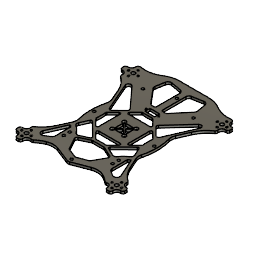
mira_main_body (Autodesk Fusion 360 design; units mm, degrees)
part number: 2026-05-12-18-13-33-373
Autodesk Fusion 360 part; units mm, degrees
(part 1 of 4)
sketch "Esboço1" plane through (0, 0, 0) normal (0, 0, 1) x (1, 0, 0)
  circle A0 centre (75, 87.5) radius 15
  arc A1 (50.5773, 27.2494) -> (51.0282, -29.3922) centre (114.8154, -0.5617) ccw
  line L0 (51.0282, -29.3922) -> (70.7852, -73.1043)
  line L1 (70.4711, 73.2) -> (50.5773, 27.2494)
  circle A2 centre (75, -87.5) radius 15
  circle A3 centre (-75, -87.5) radius 15
  line L2 (-70.4711, 73.2) -> (-50.5773, 27.2494)
  arc A4 (-51.0282, -29.3922) -> (-50.5773, 27.2494) centre (-114.8154, -0.5617) ccw
  line L3 (-51.0282, -29.3922) -> (-70.7852, -73.1043)
  circle A5 centre (-75, 87.5) radius 15
  arc A6 (46.7294, 108.889) -> (73.7447, 102.4474) centre (70.0264, 146.7235) ccw
  arc A7 (-72.6915, 102.3213) -> (-44.7852, 108.3244) centre (-66.5604, 141.6847) ccw
  line L4 (0, 0) -> (0, 132.4678) construction
  arc A8 (-23.7067, 29.0729) -> (-23.5953, 33.2362) centre (-25.8097, 31.2123) ccw
  line L5 (-23.7067, 29.0729) -> (-36.9334, 16.0716)
  arc A9 (-41.7895, 17.0192) -> (-36.9334, 16.0716) centre (-39.0364, 18.2111) ccw
  line L6 (-61.9965, 63.6935) -> (-41.7895, 17.0192)
  line L7 (-55.3948, 68.0303) -> (-23.5953, 33.2362)
  circle A10 centre (-58.3475, 65.3318) radius 4
  arc A11 (9.266, 38.142) -> (7.6383, 38.7303) centre (7.8393, 36.7404) ccw
  line L8 (9.266, 38.142) -> (19.2664, 27.9622)
  arc A12 (17.8415, 24.5606) -> (19.2664, 27.9622) centre (17.8397, 26.5606) ccw
  line L9 (17.8415, 24.5606) -> (-17.871, 24.5283)
  arc A13 (-19.3052, 27.9241) -> (-17.871, 24.5283) centre (-17.8728, 26.5283) ccw
  line L10 (-9.3455, 38.1438) -> (-19.3052, 27.9241)
  arc A14 (-7.7103, 38.7376) -> (-9.3455, 38.1438) centre (-7.9132, 36.7479) ccw
  arc A15 (-7.7103, 38.7376) -> (7.6383, 38.7303) centre (0, 114.3455) ccw
  arc A16 (23.5625, 33.2372) -> (23.6374, 29.1331) centre (25.7596, 31.2246) ccw
  line L11 (23.6374, 29.1331) -> (36.246, 16.5772)
  arc A17 (36.246, 16.5772) -> (41.8922, 17.2564) centre (38.8636, 18.6251) ccw
  line L12 (61.9967, 63.6938) -> (41.8922, 17.2564)
  line L13 (55.4143, 68.0759) -> (23.5625, 33.2372)
  circle A18 centre (58.3695, 65.3802) radius 4
  line L14 (38.1438, -9.3455) -> (27.9241, -19.3052)
  arc A19 (38.1438, -9.3455) -> (38.7376, -7.7103) centre (36.7479, -7.9132) ccw
  arc A20 (38.7303, 7.6383) -> (38.7376, -7.7103) centre (114.3455, 0) ccw
  arc A21 (38.7303, 7.6383) -> (38.142, 9.266) centre (36.7404, 7.8393) ccw
  line L15 (38.142, 9.266) -> (27.9622, 19.2664)
  arc A22 (27.9622, 19.2664) -> (24.5607, 17.8415) centre (26.5606, 17.8397) ccw
  arc A23 (24.5283, -17.871) -> (27.9241, -19.3052) centre (26.5283, -17.8728) ccw
  line L16 (24.5606, 17.8415) -> (24.5283, -17.871)
  arc A24 (19.3052, -27.9241) -> (17.871, -24.5283) centre (17.8728, -26.5283) ccw
  line L17 (9.3455, -38.1438) -> (19.3052, -27.9241)
  arc A25 (7.7103, -38.7376) -> (9.3455, -38.1438) centre (7.9132, -36.7479) ccw
  arc A26 (7.7103, -38.7376) -> (-7.6383, -38.7303) centre (0, -114.3455) ccw
  arc A27 (-9.266, -38.142) -> (-7.6383, -38.7303) centre (-7.8393, -36.7404) ccw
  line L18 (-9.266, -38.142) -> (-19.2664, -27.9622)
  arc A28 (-17.8415, -24.5606) -> (-19.2664, -27.9622) centre (-17.8397, -26.5606) ccw
  line L19 (-17.8415, -24.5606) -> (17.871, -24.5283)
  arc A29 (-27.9955, -19.2498) -> (-24.5916, -17.8264) centre (-26.5916, -17.8253) ccw
  line L20 (-38.1463, -9.2454) -> (-27.9955, -19.2498)
  arc A30 (-38.7321, -7.6192) -> (-38.1463, -9.2454) centre (-36.7424, -7.821) ccw
  arc A31 (-38.7321, -7.6192) -> (-38.7256, 7.6527) centre (-114.3432, 0.0492) ccw
  arc A32 (-38.1376, 9.2791) -> (-38.7256, 7.6527) centre (-36.7356, 7.8528) ccw
  line L21 (-38.1376, 9.2791) -> (-27.9736, 19.2699)
  arc A33 (-24.5716, 17.8424) -> (-27.9736, 19.2699) centre (-26.5716, 17.8436) ccw
  line L22 (-24.5716, 17.8424) -> (-24.5916, -17.8264)
  arc A34 (-34.7856, -45.3775) -> (-28.3187, -47.4234) centre (-30.444, -42.8975) ccw
  arc A35 (-34.7856, -45.3775) -> (-44.4886, -35.8486) centre (-56.4937, -57.7776) ccw
  arc A36 (-46.6438, -29.4035) -> (-44.4886, -35.8486) centre (-42.0875, -31.4628) ccw
  line L23 (-40.6601, -16.1647) -> (-46.6438, -29.4035)
  arc A37 (-37.4337, -15.5639) -> (-40.6601, -16.1647) centre (-38.8376, -16.9884) ccw
  line L24 (-37.4337, -15.5639) -> (-14.6425, -38.0264)
  arc A38 (-15.1963, -41.2612) -> (-14.6425, -38.0264) centre (-16.0464, -39.4508) ccw
  line L25 (-15.1963, -41.2612) -> (-28.3187, -47.4234)
  arc A39 (44.339, -36.0244) -> (34.6129, -45.4956) centre (56.2565, -57.9923) ccw
  arc A40 (44.339, -36.0244) -> (46.7322, -29.5993) centre (42.0339, -31.5075) ccw
  line L26 (40.9054, -16.7074) -> (46.7322, -29.5993)
  arc A41 (40.9054, -16.7074) -> (37.3489, -15.6517) centre (38.8619, -17.0732) ccw
  line L27 (37.3489, -15.6517) -> (14.46, -38.0146)
  arc A42 (14.46, -38.0146) -> (14.9942, -41.2515) centre (15.8549, -39.4469) ccw
  arc A43 (28.1234, -47.5076) -> (34.6129, -45.4956) centre (30.28, -42.9921) ccw
  line L28 (14.9942, -41.2515) -> (28.1234, -47.5076)
  line L29 (-9.1318, 102.3881) -> (-26.9725, 105.5339)
  arc A44 (-26.9725, 105.5339) -> (-32.7648, 101.4781) centre (-27.8408, 100.6098) ccw
  line L30 (-32.7648, 101.4781) -> (-35.4243, 86.3954)
  arc A45 (-35.4243, 86.3954) -> (-34.3305, 82.3132) centre (-30.5003, 85.5271) ccw
  line L31 (-34.3305, 82.3132) -> (-14.3032, 58.4456)
  arc A46 (-14.3032, 58.4456) -> (-10.473, 56.6595) centre (-10.473, 61.6595) ccw
  line L32 (-10.473, 56.6595) -> (-7, 56.6595)
  arc A47 (-7, 56.6595) -> (-5, 58.6595) centre (-7, 58.6595) ccw
  arc A48 (-5, 97.464) -> (-9.1318, 102.3881) centre (-10, 97.464) ccw
  line L33 (-5, 58.6595) -> (-5, 97.464)
  arc A49 (9.1318, 102.3881) -> (5, 97.464) centre (10, 97.464) ccw
  line L34 (9.1318, 102.3881) -> (26.9725, 105.5339)
  arc A50 (32.7648, 101.4781) -> (26.9725, 105.5339) centre (27.8408, 100.6098) ccw
  line L35 (32.7648, 101.4781) -> (35.4243, 86.3954)
  arc A51 (34.3305, 82.3132) -> (35.4243, 86.3954) centre (30.5003, 85.5271) ccw
  line L36 (34.3305, 82.3132) -> (14.3032, 58.4456)
  arc A52 (10.473, 56.6595) -> (14.3032, 58.4456) centre (10.473, 61.6595) ccw
  line L37 (10.473, 56.6595) -> (7, 56.6595)
  arc A53 (5, 58.6595) -> (7, 56.6595) centre (7, 58.6595) ccw
  line L38 (5, 58.6595) -> (5, 97.464)
  line L39 (0, 0) -> (0, 114.3455) construction
  line L40 (2.1213, -0.7071) -> (8.1464, -6.7322)
  line L41 (0, 0) -> (20, 0) construction
  circle A54 centre (10, 10) radius 1.5
  line L42 (-10, -10) -> (10, 10) construction
  line L43 (-2.1213, 0.7071) -> (-8.1464, 6.7322)
  arc A55 (-6.7322, -8.1464) -> (-6.3787, -9) centre (-6.3787, -8.5) ccw
  arc A56 (-6.3787, 9) -> (-6.7322, 8.1464) centre (-6.3787, 8.5) ccw
  arc A57 (-0.7071, 2.1213) -> (0.7071, 2.1213) centre (0, 2.8284) ccw
  line L44 (8.1464, 6.7322) -> (2.1213, 0.7071)
  line L45 (6.7322, -8.1464) -> (0.7071, -2.1213)
  arc A58 (6.3787, -9) -> (6.7322, -8.1464) centre (6.3787, -8.5) ccw
  line L46 (-8.1464, -6.7322) -> (-2.1213, -0.7071)
  line L47 (-10, 10) -> (10, 10)
  line L48 (-0.7071, -2.1213) -> (-6.7322, -8.1464)
  line L49 (-9, 6.3787) -> (-9, -6.3787)
  line L50 (10, -10) -> (-10, -10)
  circle A59 centre (-10, 10) radius 1.5
  line L51 (10, 10) -> (10, -10)
  arc A60 (6.7322, 8.1464) -> (6.3787, 9) centre (6.3787, 8.5) ccw
  arc A61 (9, 6.3787) -> (8.1464, 6.7322) centre (8.5, 6.3787) ccw
  arc A62 (0.7071, -2.1213) -> (-0.7071, -2.1213) centre (0, -2.8284) ccw
  arc A63 (2.1213, 0.7071) -> (2.1213, -0.7071) centre (2.8284, 0) ccw
  arc A64 (-2.1213, -0.7071) -> (-2.1213, 0.7071) centre (-2.8284, 0) ccw
  arc A65 (8.1464, -6.7322) -> (9, -6.3787) centre (8.5, -6.3787) ccw
  circle A66 centre (10, -10) radius 1.5
  arc A67 (-9, -6.3787) -> (-8.1464, -6.7322) centre (-8.5, -6.3787) ccw
  line L52 (-10, -10) -> (-10, 10)
  line L53 (-6.3787, -9) -> (6.3787, -9)
  line L54 (10, -10) -> (-10, 10) construction
  line L55 (-6.7322, 8.1464) -> (-0.7071, 2.1213)
  line L56 (0.7071, 2.1213) -> (6.7322, 8.1464)
  line L57 (9, -6.3787) -> (9, 6.3787)
  circle A68 centre (-10, -10) radius 1.5
  line L58 (6.3787, 9) -> (-6.3787, 9)
  arc A69 (-8.1464, 6.7322) -> (-9, 6.3787) centre (-8.5, 6.3787) ccw
  circle A70 centre (0, -87.5) radius 6
  line L59 (0, -87.5) -> (0, -54) construction
  line L60 (0, -81.5) -> (-15.6612, -75.3836)
  line L61 (0, -81.5) -> (16.4256, -75.2214)
  line L62 (2.1423, -93.1045) -> (36.9275, -79.8081)
  line L63 (-2.1827, -93.0889) -> (-35.9657, -79.8952)
  arc A71 (-35.9657, -79.8952) -> (-60.1979, -89.9288) centre (0.31, -201.7835) ccw
  arc A72 (60.2098, -89.9999) -> (36.9275, -79.8081) centre (-2.2046, -200.8918) ccw
  circle A73 centre (0, -87.5) radius 2.15
  line L64 (-26.2105, -50.915) -> (-10.6059, -43.5872)
  line L65 (-9.3307, -43.3027) -> (9.3218, -43.3027)
  line L66 (10.6123, -43.5944) -> (26.8632, -51.3381)
  line L67 (28.1945, -55.5044) -> (17.9762, -73.8773)
  line L68 (-17.2021, -74.0283) -> (-27.5676, -55.0697)
  arc A74 (-26.2105, -50.915) -> (-27.5676, -55.0697) centre (-24.9353, -53.6305) ccw
  arc A75 (-9.3307, -43.3027) -> (-10.6059, -43.5872) centre (-9.3307, -46.3027) ccw
  arc A76 (10.6123, -43.5944) -> (9.3218, -43.3027) centre (9.3218, -46.3027) ccw
  arc A77 (28.1945, -55.5044) -> (26.8632, -51.3381) centre (25.5727, -54.0463) ccw
  arc A78 (16.4256, -75.2214) -> (17.9762, -73.8773) centre (15.3544, -72.4192) ccw
  arc A79 (-17.2021, -74.0283) -> (-15.6612, -75.3836) centre (-14.5698, -72.5892) ccw
  line L69 (25.7561, 114.8285) -> (-22.9214, 114.8285)
  arc A80 (46.7294, 108.889) -> (25.7561, 114.8285) centre (25.7561, 74.8285) ccw
  arc A81 (-22.9214, 114.8285) -> (-44.7852, 108.3244) centre (-22.9214, 74.8285) ccw
  point P0 (9, 7.5858)
  point P1 (9, -7.5858)
  point P2 (-10, -43.3027)
  point P3 (10, -43.3027)
  dimension "d1" = 30
  dimension "d2" = 30
  dimension "d3" = 30
  dimension "d4" = 30
  dimension "d5" = 127.25
  dimension "d6" = 70
  dimension "d9" = 150
  dimension "d10" = 150
  dimension "d11" = 8
  dimension "d12" = 3
  dimension "d13" = 4
  dimension "d14" = 2
  dimension "d15" = 4
  dimension "d16" = 2
  dimension "d17" = 69.738
  dimension "d18" = 69.738
  dimension "d19" = 32
  dimension "d20" = 25
  dimension "d21" = 5
  dimension "d22" = 4
  dimension "d23" = 4
  dimension "d24" = 4
  dimension "d25" = 4
  dimension "d26" = 130
  dimension "d27" = 100
  dimension "d28" = 5
  dimension "d29" = 2
  dimension "d30" = 38.8045
  dimension "d31" = 31.1569
  dimension "d32" = 15.0827
  dimension "d33" = 17.8408
  dimension "d34" = 5
  dimension "d35" = 100
  dimension "d36" = 2
  dimension "d37" = 5
  dimension "d38" = 3.473
  dimension "d39" = 31.1569
  dimension "d40" = 38.8045
  dimension "d41" = 17.8408
  dimension "d42" = 5
  dimension "d43" = 15.0827
  dimension "d44" = 5
  dimension "d45" = 5
  dimension "d62" = 360
  dimension "d63" = 3
  dimension "d64" = 3
  dimension "d65" = 3
  dimension "d66" = 3
  dimension "d67" = 1
  dimension "d68" = 1
  dimension "d69" = 1
  dimension "d70" = 0.5
  dimension "d71" = 20
  dimension "d72" = 20
  dimension "d73" = 1
  dimension "d149" = 12
  dimension "d150" = 87.5
  dimension "d153" = 4.3
  dimension "d166" = 140
  dimension "d167" = 140
  dimension "d168" = 20
  dimension "d169" = 4
  dimension "d170" = 3
  dimension "d171" = 40
  dimension "d173" = 87.5
  dimension "d186" = 87.5
  dimension "d187" = 87.5
  dimension "d188" = 87.5
  dimension "d189" = 75
  dimension "d190" = 75
  constraint coincident L2.start A5
  constraint coincident L3.end A3
  constraint coincident A72.start A2
  constraint coincident A71.end A3
  constraint tangent L2 A4
  constraint tangent A4 L3
  constraint tangent A1 L1
  constraint tangent A1 L0
  constraint equal A1 A4
  constraint coincident L1.start A0
  constraint equal L1 L2
  constraint equal L0 L3
  constraint coincident A7.start A5
  constraint coincident A6.end A0
  constraint tangent A5 A7
  constraint tangent A0 A6
  constraint coincident L4.start L39.start
  constraint symmetric A0 A5 L4
  constraint symmetric A2 A3 L4
  constraint symmetric A1 A4 L4
  constraint coincident L6.start A10
  constraint coincident L7.start A10
  constraint tangent A9 L6
  constraint tangent L5 A9
  constraint tangent A8 L7
  constraint tangent A8 L5
  constraint equal A8 A9
  constraint tangent L7 A10
  constraint parallel L5 L21
  constraint tangent L21 A33
  constraint tangent A33 L22
  constraint tangent A29 L20
  constraint tangent A29 L22
  constraint equal A29 A33
  constraint tangent L20 A30
  constraint tangent A30 A31
  constraint equal A30 A33
  constraint tangent A32 L21
  constraint tangent A31 A32
  constraint equal A32 A33
  constraint equal L20 L21
  constraint parallel L20 L24
  constraint tangent A37 L24
  constraint tangent L23 A37
  constraint tangent L24 A38
  constraint tangent A38 L25
  constraint equal A37 A38
  constraint tangent A34 L25
  constraint tangent A34 A35
  constraint tangent A36 L23
  constraint tangent A35 A36
  constraint equal A34 A36
  constraint perpendicular L32 L33
  constraint perpendicular L29 L30
  constraint tangent A44 L30
  constraint tangent L29 A44
  constraint tangent A48 L33
  constraint tangent L29 A48
  constraint equal A44 A48
  constraint tangent L30 A45
  constraint tangent A45 L31
  constraint equal A44 A45
  constraint tangent L31 A46
  constraint tangent A46 L32
  constraint equal A44 A46
  constraint tangent L32 A47
  constraint tangent A47 L33
  constraint coincident A15.centre L39.end
  constraint coincident L0.end A2
  constraint coincident L13.start A18
  constraint coincident L12.start A18
  constraint horizontal L50
  constraint perpendicular L50 L52
  constraint parallel L47 L50
  constraint parallel L51 L52
  constraint coincident L4.start L54
  constraint coincident L4.start L42
  constraint coincident L50.start L51.end
  constraint coincident L42.start L50.end
  constraint coincident A54.centre L42.end
  constraint coincident L47.start A59.centre
  constraint parallel L51 L57
  constraint parallel L40 L54
  constraint parallel L42 L44
  constraint perpendicular L41 L57
  constraint coincident P1 L57
  constraint coincident P1 L40
  constraint tangent A65 L57
  constraint tangent L40 A65
  constraint coincident P0 L57
  constraint coincident P0 L44
  constraint tangent A61 L57
  constraint tangent L44 A61
  constraint equal A61 A65
  constraint tangent L44 A63
  constraint tangent L40 A63
  constraint coincident A70.centre L59.start
  constraint vertical L59
  constraint coincident A70 L60.start
  constraint coincident L59 L60.start
  constraint coincident A70 L62.start
  constraint coincident A70 L63.start
  constraint tangent A70 L63
  constraint tangent A70 L62
  constraint parallel L60 L63
  constraint parallel L61 L62
  constraint concentric A70 A73
  constraint horizontal L65
  constraint parallel L25 L64
  constraint parallel L28 L66
  constraint symmetric L59 P2 P3
  constraint tangent L64 A74
  constraint tangent L68 A74
  constraint coincident P2 L64
  constraint tangent L64 A75
  constraint tangent L65 A75
  constraint equal A74 A75
  constraint coincident P3 L65
  constraint coincident P3 L66
  constraint tangent L65 A76
  constraint tangent L66 A76
  constraint equal A74 A76
  constraint tangent L66 A77
  constraint tangent L67 A77
  constraint equal A74 A77
  constraint tangent L61 A78
  constraint tangent L67 A78
  constraint equal A74 A78
  constraint tangent L60 A79
  constraint tangent L68 A79
  constraint equal A74 A79
  constraint perpendicular L4 L69
  constraint tangent L69 A80
  constraint tangent A6 A80
  constraint tangent L69 A81
  constraint tangent A7 A81
  constraint equal A80 A81
  measures "d1" diameter of A5
  measures "d2" diameter of A0
  measures "d3" diameter of A3
  measures "d4" diameter of A2
  measures "d5" radius of A72
  measures "d6" radius of A4
  measures "d9" distance of A3.centre A2.centre
  measures "d10" distance of A5.centre A0.centre
  measures "d11" diameter of A10
  measures "d12" radius of A9
  measures "d13" distance of L5 L21
  measures "d14" radius of A33
  measures "d15" distance of L20 L24
  measures "d16" radius of A37
  measures "d17" angle of L23 L24
  measures "d18" angle of L24 L25
  measures "d19" distance of L24.end A37.start
  measures "d20" radius of A35
  measures "d21" radius of A34
  measures "d22" distance of L2 L6
  measures "d23" distance of L1 L12
  measures "d24" distance of L0 L26
  measures "d25" distance of L3 L23
  measures "d26" angle of L31 L32
  measures "d27" angle of L29 L33
  measures "d28" radius of A44
  measures "d29" radius of A47
  measures "d30" distance of A48.start A47.end
  measures "d31" distance of L31.end A45.end
  measures "d32" vertical distance of A44.end L30.end
  measures "d33" horizontal distance of L29.start L29.end
  measures "d34" distance of L33 L39
  measures "d35" angle of L34 L38
  measures "d36" radius of A53
  measures "d37" radius of A52
  measures "d38" distance of A52.start L37.end
  measures "d39" distance of A51.start L36.end
  measures "d40" distance of A49.end A53.start
  measures "d41" horizontal distance of A49.start L34.end
  measures "d42" radius of A50
  measures "d43" vertical distance of L35.end A50.start
  measures "d44" radius of A51
  measures "d45" distance of L38 L39
  measures "d63" diameter of A66
  measures "d64" diameter of A68
  measures "d65" diameter of A54
  measures "d66" diameter of A59
  measures "d67" distance of L51 L57
  measures "d68" distance of L42 L44
  measures "d69" distance of L40 L54
  measures "d70" radius of A65
  measures "d71" distance of L50.start A54.centre
  measures "d72" distance of L42.start L50.start
  measures "d73" radius of A63
  measures "d149" diameter of A70
  measures "d150" distance of L4.start A70.centre
  measures "d153" diameter of A73
  measures "d166" angle of L61 L67
  measures "d167" angle of L60 L68
  measures "d168" distance of P2 P3
  measures "d169" distance of L28 L66
  measures "d170" radius of A74
  measures "d171" radius of A80
  measures "d173" vertical distance of A2.centre L4.start
  measures "d186" vertical distance of A0.centre L4.start
  measures "d187" vertical distance of A5.centre L4.start
  measures "d188" vertical distance of A3.centre L4.start
  measures "d189" horizontal distance of L4.start A3.centre
  measures "d190" horizontal distance of A0.centre L4.start
extrude "Extrusão1" add sketch "Esboço1" along normal mid plane 4 contours A0 | A0 A1 L0 L1 A2 A3 L2 A4 L3 A5 A6 A7 A70 L62 L63 A71 A72 L69 A80 A81 | A2 | A5 | A70 | A3 | A54 L47 L51 | A54 L47 L51 | A54 L47 L50 A59 L51 A66 L52 A68 | L47 A59 L52 | L47 A59 L52 | L50 L51 A66 | L50 L51 A66 | L50 L52 A68 | L50 L52 A68
sketch "Esboço2" plane through (0, 0, 2) normal (0, 0, 1) x (-1, 0, 0)
  line L0 (14.9943, 41.2512) -> (28.1237, 47.5069)
  line L1 (49.5538, 39.7214) -> (47.4521, 41.7697)
  arc A0 (47.15, 42.4858) -> (47.4521, 41.7697) centre (48.15, 42.4858) ccw
  arc A1 (49.5538, 39.7214) -> (51.1653, 40.0309) centre (50.2517, 40.4376) ccw
  line L2 (47.15, 42.4858) -> (47.15, 67.561)
  arc A2 (49.4611, 71.7764) -> (47.15, 67.561) centre (52.15, 67.561) ccw
  arc A3 (-14.4588, 38.0133) -> (-14.9943, 41.2512) centre (-15.8546, 39.4456) ccw
  arc A4 (-47.15, 67.561) -> (-49.4611, 71.7764) centre (-52.15, 67.561) ccw
  circle A5 centre (-40.65, 60) radius 2.15
  arc A6 (-24.5283, 17.871) -> (-27.9241, 19.3052) centre (-26.5283, 17.8728) ccw
  arc A7 (-47.4521, 41.7697) -> (-47.15, 42.4858) centre (-48.15, 42.4858) ccw
  line L3 (-47.15, 42.4858) -> (-47.15, 67.561)
  line L4 (-28.1237, 47.5069) -> (-14.9943, 41.2512)
  line L5 (-32.8675, 14.4875) -> (-27.9241, 19.3052)
  line L6 (-49.4611, 71.7764) -> (-57.5607, 76.943)
  arc A8 (14.9943, 41.2512) -> (14.4588, 38.0133) centre (15.8546, 39.4456) ccw
  arc A9 (34.6056, 45.4913) -> (44.3323, 36.0121) centre (56.2613, 57.9825) ccw
  line L7 (-49.5538, 39.7214) -> (-47.4521, 41.7697)
  arc A10 (-40.5988, 16.2982) -> (-37.3758, 15.6793) centre (-38.7717, 17.1116) ccw
  arc A11 (-57.5607, 76.943) -> (-64.8173, 70.6939) centre (-60.2496, 72.7276) ccw
  arc A12 (-28.1237, 47.5069) -> (-34.6056, 45.4913) centre (-30.2744, 42.9931) ccw
  line L8 (-14.4588, 38.0133) -> (-15.8157, 36.6909)
  line L9 (17.8415, 24.5606) -> (-17.871, 24.5283)
  circle A13 centre (-40.65, 50) radius 2.15
  line L10 (-19.3052, 27.9241) -> (-9.3455, 38.1438)
  arc A14 (-7.7103, 38.7376) -> (-9.3455, 38.1438) centre (-7.9132, 36.7479) ccw
  arc A15 (-7.7103, 38.7376) -> (7.6383, 38.7303) centre (0, 114.3455) ccw
  arc A16 (-19.3052, 27.9241) -> (-17.871, 24.5283) centre (-17.8728, 26.5283) ccw
  arc A17 (-51.1653, 40.0309) -> (-49.5538, 39.7214) centre (-50.2517, 40.4376) ccw
  circle A18 centre (40.65, 50) radius 2.15
  circle A19 centre (40.65, 60) radius 2.15
  line L11 (49.4611, 71.7764) -> (57.5607, 76.943)
  arc A20 (34.6056, 45.4913) -> (28.1237, 47.5069) centre (30.2744, 42.9931) ccw
  arc A21 (9.266, 38.142) -> (7.6383, 38.7303) centre (7.8393, 36.7404) ccw
  arc A22 (-38.1438, 9.3455) -> (-38.7376, 7.7103) centre (-36.7479, 7.9132) ccw
  arc A23 (64.8173, 70.6939) -> (57.5607, 76.943) centre (60.2496, 72.7276) ccw
  line L12 (51.1653, 40.0309) -> (64.8173, 70.6939)
  arc A24 (-38.7376, -7.7103) -> (-38.7303, -7.6383) centre (-114.3455, 0) ccw
  arc A25 (46.5142, 29.5844) -> (44.3323, 36.0121) centre (41.9465, 31.618) ccw
  line L13 (-51.1653, 40.0309) -> (-64.8173, 70.6939)
  line L14 (0, 38.3455) -> (0, 95) construction
  line L15 (19.3052, -27.9241) -> (9.3455, -38.1438)
  arc A26 (7.7103, -38.7376) -> (9.3455, -38.1438) centre (7.9132, -36.7479) ccw
  arc A27 (7.7103, -38.7376) -> (-7.6383, -38.7303) centre (0, -114.3455) ccw
  arc A28 (-9.266, -38.142) -> (-7.6383, -38.7303) centre (-7.8393, -36.7404) ccw
  line L16 (-9.266, -38.142) -> (-19.2664, -27.9622)
  arc A29 (-17.8415, -24.5606) -> (-19.2664, -27.9622) centre (-17.8397, -26.5606) ccw
  line L17 (-17.8415, -24.5606) -> (17.871, -24.5283)
  arc A30 (19.3052, -27.9241) -> (17.871, -24.5283) centre (17.8728, -26.5283) ccw
  line L18 (70.4711, -73.2) -> (50.5773, -27.2494)
  arc A31 (51.0282, 29.3922) -> (50.5773, -27.2494) centre (114.8154, 0.5617) ccw
  line L19 (51.0282, 29.3922) -> (70.7852, 73.1043)
  arc A32 (70.7852, 73.1043) -> (60.1979, 89.9288) centre (75, 87.5) ccw
  arc A33 (35.9657, 79.8952) -> (60.1979, 89.9288) centre (-0.31, 201.7835) ccw
  arc A34 (-60.2098, 89.9999) -> (-70.7852, 73.1043) centre (-75, 87.5) ccw
  line L20 (-70.7852, 73.1043) -> (-51.0282, 29.3922)
  arc A35 (-50.5773, -27.2494) -> (-51.0282, 29.3922) centre (-114.8154, 0.5617) ccw
  line L21 (-50.5773, -27.2494) -> (-70.4711, -73.2)
  arc A36 (-70.4711, -73.2) -> (-73.7447, -102.4474) centre (-75, -87.5) ccw
  arc A37 (-46.7294, -108.889) -> (-73.7447, -102.4474) centre (-70.0264, -146.7235) ccw
  arc A38 (72.6915, -102.3213) -> (44.7852, -108.3244) centre (66.5604, -141.6847) ccw
  arc A39 (72.6915, -102.3213) -> (70.4711, -73.2) centre (75, -87.5) ccw
  arc A40 (38.1376, -9.2791) -> (38.7256, -7.6527) centre (36.7356, -7.8528) ccw
  line L22 (38.1376, -9.2791) -> (27.9736, -19.2699)
  arc A41 (24.5716, -17.8424) -> (27.9736, -19.2699) centre (26.5716, -17.8436) ccw
  line L23 (24.5716, -17.8424) -> (24.5916, 17.8264)
  arc A42 (27.9955, 19.2498) -> (24.5916, 17.8264) centre (26.5916, 17.8253) ccw
  line L24 (27.9955, 19.2498) -> (38.1463, 9.2454)
  arc A43 (38.7321, 7.6192) -> (38.1463, 9.2454) centre (36.7424, 7.821) ccw
  arc A44 (38.7321, 7.6192) -> (38.7256, -7.6527) centre (114.3432, -0.0492) ccw
  arc A45 (-10.473, -56.6595) -> (-14.3032, -58.4456) centre (-10.473, -61.6595) ccw
  line L25 (-10.473, -56.6595) -> (-7, -56.6595)
  arc A46 (-5, -58.6595) -> (-7, -56.6595) centre (-7, -58.6595) ccw
  line L26 (-5, -58.6595) -> (-5, -97.464)
  arc A47 (-9.1318, -102.3881) -> (-5, -97.464) centre (-10, -97.464) ccw
  line L27 (-9.1318, -102.3881) -> (-26.9725, -105.5339)
  arc A48 (-32.7648, -101.4781) -> (-26.9725, -105.5339) centre (-27.8408, -100.6098) ccw
  line L28 (-32.7648, -101.4781) -> (-35.4243, -86.3954)
  arc A49 (-34.3305, -82.3132) -> (-35.4243, -86.3954) centre (-30.5003, -85.5271) ccw
  line L29 (-34.3305, -82.3132) -> (-14.3032, -58.4456)
  line L30 (5, -97.464) -> (5, -58.6595)
  arc A50 (7, -56.6595) -> (5, -58.6595) centre (7, -58.6595) ccw
  line L31 (7, -56.6595) -> (10.473, -56.6595)
  arc A51 (14.3032, -58.4456) -> (10.473, -56.6595) centre (10.473, -61.6595) ccw
  line L32 (14.3032, -58.4456) -> (34.3305, -82.3132)
  arc A52 (35.4243, -86.3954) -> (34.3305, -82.3132) centre (30.5003, -85.5271) ccw
  line L33 (35.4243, -86.3954) -> (32.7648, -101.4781)
  arc A53 (26.9725, -105.5339) -> (32.7648, -101.4781) centre (27.8408, -100.6098) ccw
  line L34 (26.9725, -105.5339) -> (9.1318, -102.3881)
  arc A54 (5, -97.464) -> (9.1318, -102.3881) centre (10, -97.464) ccw
  arc A55 (-38.7303, -7.6383) -> (-38.142, -9.266) centre (-36.7404, -7.8393) ccw
  arc A56 (-38.7303, -7.6383) -> (-38.7376, 7.7103) centre (-114.3455, 0) ccw
  arc A57 (-38.1438, 9.3455) -> (-38.7376, 7.7103) centre (-36.7479, 7.9132) ccw
  line L35 (-38.1438, 9.3455) -> (-27.9241, 19.3052)
  arc A58 (-24.5283, 17.871) -> (-27.9241, 19.3052) centre (-26.5283, 17.8728) ccw
  line L36 (-24.5283, 17.871) -> (-24.5606, -17.8415)
  arc A59 (-27.9622, -19.2664) -> (-24.5607, -17.8415) centre (-26.5606, -17.8397) ccw
  line L37 (-27.9622, -19.2664) -> (-38.142, -9.266)
  arc A60 (37.4337, 15.5639) -> (40.6601, 16.1647) centre (38.8376, 16.9884) ccw
  line L38 (37.4337, 15.5639) -> (14.6425, 38.0264)
  arc A61 (15.1963, 41.2612) -> (14.6425, 38.0264) centre (16.0464, 39.4508) ccw
  line L39 (15.1963, 41.2612) -> (28.3187, 47.4234)
  arc A62 (34.7856, 45.3775) -> (28.3187, 47.4234) centre (30.444, 42.8975) ccw
  arc A63 (34.7856, 45.3775) -> (44.4886, 35.8486) centre (56.4937, 57.7776) ccw
  arc A64 (46.6438, 29.4035) -> (44.4886, 35.8486) centre (42.0875, 31.4628) ccw
  line L40 (46.6438, 29.4035) -> (40.6601, 16.1647)
  line L41 (41.7895, -17.0192) -> (61.9965, -63.6935)
  arc A65 (55.3948, -68.0303) -> (61.9965, -63.6935) centre (58.3475, -65.3318) ccw
  line L42 (55.3948, -68.0303) -> (23.5953, -33.2362)
  arc A66 (23.7067, -29.0729) -> (23.5953, -33.2362) centre (25.8097, -31.2123) ccw
  line L43 (23.7067, -29.0729) -> (36.9334, -16.0716)
  arc A67 (41.7895, -17.0192) -> (36.9334, -16.0716) centre (39.0364, -18.2111) ccw
  arc A68 (9.266, 38.142) -> (7.6383, 38.7303) centre (7.8393, 36.7404) ccw
  line L44 (9.266, 38.142) -> (19.2664, 27.9622)
  arc A69 (17.8415, 24.5606) -> (19.2664, 27.9622) centre (17.8397, 26.5606) ccw
  line L45 (17.8415, 24.5606) -> (-17.871, 24.5283)
  arc A70 (-19.3052, 27.9241) -> (-17.871, 24.5283) centre (-17.8728, 26.5283) ccw
  line L46 (-19.3052, 27.9241) -> (-9.3455, 38.1438)
  arc A71 (-7.7103, 38.7376) -> (-9.3455, 38.1438) centre (-7.9132, 36.7479) ccw
  arc A72 (-7.7103, 38.7376) -> (7.6383, 38.7303) centre (0, 114.3455) ccw
  arc A73 (-40.9054, 16.7074) -> (-37.3489, 15.6517) centre (-38.8619, 17.0732) ccw
  line L47 (-40.9054, 16.7074) -> (-46.7322, 29.5993)
  arc A74 (-44.339, 36.0244) -> (-46.7322, 29.5993) centre (-42.0339, 31.5075) ccw
  arc A75 (-44.339, 36.0244) -> (-34.6129, 45.4956) centre (-56.2565, 57.9923) ccw
  arc A76 (-28.1234, 47.5076) -> (-34.6129, 45.4956) centre (-30.28, 42.9921) ccw
  line L48 (-28.1234, 47.5076) -> (-14.9942, 41.2515)
  arc A77 (-14.46, 38.0146) -> (-14.9942, 41.2515) centre (-15.8549, 39.4469) ccw
  line L49 (-14.46, 38.0146) -> (-37.3489, 15.6517)
  arc A78 (-61.9967, -63.6938) -> (-55.4143, -68.0759) centre (-58.3695, -65.3802) ccw
  line L50 (-61.9967, -63.6938) -> (-41.8922, -17.2564)
  arc A79 (-36.246, -16.5772) -> (-41.8922, -17.2564) centre (-38.8636, -18.6251) ccw
  line L51 (-36.246, -16.5772) -> (-23.6374, -29.1331)
  arc A80 (-23.5625, -33.2372) -> (-23.6374, -29.1331) centre (-25.7596, -31.2246) ccw
  line L52 (-23.5625, -33.2372) -> (-55.4143, -68.0759)
  line L53 (8.1464, -6.7322) -> (2.1213, -0.7071)
  arc A81 (2.1213, 0.7071) -> (2.1213, -0.7071) centre (2.8284, 0) ccw
  line L54 (2.1213, 0.7071) -> (8.1464, 6.7322)
  arc A82 (9, 6.3787) -> (8.1464, 6.7322) centre (8.5, 6.3787) ccw
  line L55 (9, 6.3787) -> (9, -6.3787)
  arc A83 (8.1464, -6.7322) -> (9, -6.3787) centre (8.5, -6.3787) ccw
  arc A84 (-6.7322, -8.1464) -> (-6.3787, -9) centre (-6.3787, -8.5) ccw
  line L56 (-6.7322, -8.1464) -> (-0.7071, -2.1213)
  arc A85 (0.7071, -2.1213) -> (-0.7071, -2.1213) centre (0, -2.8284) ccw
  line L57 (0.7071, -2.1213) -> (6.7322, -8.1464)
  arc A86 (6.3787, -9) -> (6.7322, -8.1464) centre (6.3787, -8.5) ccw
  line L58 (6.3787, -9) -> (-6.3787, -9)
  arc A87 (-8.1464, 6.7322) -> (-9, 6.3787) centre (-8.5, 6.3787) ccw
  line L59 (-8.1464, 6.7322) -> (-2.1213, 0.7071)
  arc A88 (-2.1213, -0.7071) -> (-2.1213, 0.7071) centre (-2.8284, 0) ccw
  line L60 (-2.1213, -0.7071) -> (-8.1464, -6.7322)
  arc A89 (-9, -6.3787) -> (-8.1464, -6.7322) centre (-8.5, -6.3787) ccw
  line L61 (-9, -6.3787) -> (-9, 6.3787)
  arc A90 (6.7322, 8.1464) -> (6.3787, 9) centre (6.3787, 8.5) ccw
  line L62 (6.7322, 8.1464) -> (0.7071, 2.1213)
  arc A91 (-0.7071, 2.1213) -> (0.7071, 2.1213) centre (0, 2.8284) ccw
  line L63 (-0.7071, 2.1213) -> (-6.7322, 8.1464)
  arc A92 (-6.3787, 9) -> (-6.7322, 8.1464) centre (-6.3787, 8.5) ccw
  line L64 (-6.3787, 9) -> (6.3787, 9)
  line L65 (35.9657, 79.8952) -> (2.1827, 93.0889)
  arc A93 (2.1827, 93.0889) -> (-2.1423, 93.1045) centre (0, 87.5) ccw
  line L66 (0, 81.5) -> (15.6612, 75.3836)
  line L67 (-16.4256, 75.2214) -> (0, 81.5)
  line L68 (-2.1423, 93.1045) -> (-36.9275, 79.8081)
  arc A94 (-60.2098, 89.9999) -> (-36.7745, 80.3179) centre (-0.31, 201.7835) ccw
  circle A95 centre (0, 87.5) radius 2.15
  arc A96 (26.2105, 50.915) -> (27.5676, 55.0697) centre (24.9353, 53.6305) ccw
  line L69 (26.2105, 50.915) -> (10.6059, 43.5872)
  arc A97 (9.3307, 43.3027) -> (10.6059, 43.5872) centre (9.3307, 46.3027) ccw
  line L70 (9.3307, 43.3027) -> (-9.3218, 43.3027)
  arc A98 (-10.6123, 43.5944) -> (-9.3218, 43.3027) centre (-9.3218, 46.3027) ccw
  line L71 (-10.6123, 43.5944) -> (-26.8632, 51.3381)
  arc A99 (-28.1945, 55.5044) -> (-26.8632, 51.3381) centre (-25.5727, 54.0463) ccw
  line L72 (-28.1945, 55.5044) -> (-17.9762, 73.8773)
  arc A100 (-16.4256, 75.2214) -> (-17.9762, 73.8773) centre (-15.3544, 72.4192) ccw
  arc A101 (17.2021, 74.0283) -> (15.6612, 75.3836) centre (14.5698, 72.5892) ccw
  line L73 (17.2021, 74.0283) -> (27.5676, 55.0697)
  arc A102 (-46.7294, -108.889) -> (-25.7561, -114.8285) centre (-25.7561, -74.8285) ccw
  line L74 (-25.7561, -114.8285) -> (22.9214, -114.8285)
  arc A103 (22.9214, -114.8285) -> (44.7852, -108.3244) centre (22.9214, -74.8285) ccw
  point P0 (50.5815, 38.7198)
  point P1 (0.156, 201.9423)
  point P2 (0.2929, 201.9885)
  point P3 (0.2929, 201.9885)
  point P4 (2.2046, 200.8918)
  point P5 (2.2046, 200.8918)
  dimension "d48" = 4.3
  dimension "d49" = 4.3
  dimension "d50" = 10
  dimension "d51" = 40.65
  dimension "d52" = 45
  dimension "d53" = 10
  dimension "d54" = 35
  dimension "d55" = 6.5
  dimension "d56" = 1
  dimension "d57" = 5
  constraint symmetric A13 A18 L14
  constraint symmetric A5 A19 L14
  constraint tangent L12 A25
  constraint tangent A23 L12
  constraint tangent L11 A23
  constraint parallel L2 L14
  constraint coincident P0 L12
  constraint coincident P0 L1
  constraint tangent A1 L12
  constraint tangent L1 A1
  constraint tangent L1 A0
  constraint tangent A0 L2
  constraint equal A0 A1
  constraint tangent A2 L11
  constraint tangent L2 A2
  constraint symmetric A11.end A23.start L14
  constraint symmetric L11.end L6.end L14
  constraint symmetric A1.end A17.start L14
  constraint symmetric L1.start L7.start L14
  constraint symmetric A1 A17 L14
  constraint symmetric L1.end A7.start L14
  constraint symmetric A0.start A7.end L14
  constraint symmetric A0 A7 L14
  constraint symmetric A4.end A2.start L14
  constraint symmetric A4.start L2.end L14
  constraint symmetric A2 A4 L14
  constraint symmetric A11 A23 L14
  measures "d6" radius of A15.end
  measures "d48" diameter of A18
  measures "d49" diameter of A19
  measures "d50" distance of A19.centre A18.centre
  measures "d51" distance of A18.centre L14
  measures "d52" distance of A25.start A23.start
  measures "d53" diameter of A23
  measures "d54" distance of P0 A23.start
  measures "d55" distance of A18.centre L2
  measures "d56" radius of A1
  measures "d57" radius of A2
extrude "Extrusão2" cut sketch "Esboço2" against normal through all contours L1 A0 A1 L2 A2 L11 A23 L12 | A4 A7 L3 L6 L7 A11 A17 L13 | A5 | A13 | A18 | A19
sketch "Esboço13" plane through (0, 0, 2) normal (0, 0, 1) x (-1, 0, 0)
  circle A0 centre (0, 87.5) radius 2.15
  arc A1 (26.2105, 50.915) -> (27.5676, 55.0697) centre (24.9353, 53.6305) ccw
  line L0 (26.2105, 50.915) -> (10.6059, 43.5872)
  arc A2 (9.3307, 43.3027) -> (10.6059, 43.5872) centre (9.3307, 46.3027) ccw
  line L1 (9.3307, 43.3027) -> (-9.3218, 43.3027)
  arc A3 (-10.6123, 43.5944) -> (-9.3218, 43.3027) centre (-9.3218, 46.3027) ccw
  line L2 (-10.6123, 43.5944) -> (-26.8632, 51.3381)
  arc A4 (-28.1945, 55.5044) -> (-26.8632, 51.3381) centre (-25.5727, 54.0463) ccw
  line L3 (-28.1945, 55.5044) -> (-17.9762, 73.8773)
  arc A5 (-16.4256, 75.2214) -> (-17.9762, 73.8773) centre (-15.3544, 72.4192) ccw
  line L4 (-16.4256, 75.2214) -> (0, 81.5)
  line L5 (0, 81.5) -> (15.6612, 75.3836)
  arc A6 (17.2021, 74.0283) -> (15.6612, 75.3836) centre (14.5698, 72.5892) ccw
  line L6 (17.2021, 74.0283) -> (27.5676, 55.0697)
  line L7 (19.3052, -27.9241) -> (9.3455, -38.1438)
  arc A7 (7.7103, -38.7376) -> (9.3455, -38.1438) centre (7.9132, -36.7479) ccw
  arc A8 (7.7103, -38.7376) -> (-7.6383, -38.7303) centre (0, -114.3455) ccw
  arc A9 (-9.266, -38.142) -> (-7.6383, -38.7303) centre (-7.8393, -36.7404) ccw
  line L8 (-9.266, -38.142) -> (-19.2664, -27.9622)
  arc A10 (-17.8415, -24.5606) -> (-19.2664, -27.9622) centre (-17.8397, -26.5606) ccw
  line L9 (-17.8415, -24.5606) -> (17.871, -24.5283)
  arc A11 (19.3052, -27.9241) -> (17.871, -24.5283) centre (17.8728, -26.5283) ccw
  arc A12 (8.1464, -6.7322) -> (9, -6.3787) centre (8.5, -6.3787) ccw
  line L10 (8.1464, -6.7322) -> (2.1213, -0.7071)
  arc A13 (2.1213, 0.7071) -> (2.1213, -0.7071) centre (2.8284, 0) ccw
  line L11 (2.1213, 0.7071) -> (8.1464, 6.7322)
  arc A14 (9, 6.3787) -> (8.1464, 6.7322) centre (8.5, 6.3787) ccw
  line L12 (9, 6.3787) -> (9, -6.3787)
  arc A15 (38.1376, -9.2791) -> (38.7256, -7.6527) centre (36.7356, -7.8528) ccw
  line L13 (38.1376, -9.2791) -> (27.9736, -19.2699)
  arc A16 (24.5716, -17.8424) -> (27.9736, -19.2699) centre (26.5716, -17.8436) ccw
  line L14 (24.5716, -17.8424) -> (24.5916, 17.8264)
  arc A17 (27.9955, 19.2498) -> (24.5916, 17.8264) centre (26.5916, 17.8253) ccw
  line L15 (27.9955, 19.2498) -> (38.1463, 9.2454)
  arc A18 (38.7321, 7.6192) -> (38.1463, 9.2454) centre (36.7424, 7.821) ccw
  arc A19 (38.7321, 7.6192) -> (38.7256, -7.6527) centre (114.3432, -0.0492) ccw
  line L16 (-9, -6.3787) -> (-9, 6.3787)
  arc A20 (-8.1464, 6.7322) -> (-9, 6.3787) centre (-8.5, 6.3787) ccw
  line L17 (-8.1464, 6.7322) -> (-2.1213, 0.7071)
  arc A21 (-2.1213, -0.7071) -> (-2.1213, 0.7071) centre (-2.8284, 0) ccw
  line L18 (-2.1213, -0.7071) -> (-8.1464, -6.7322)
  arc A22 (-9, -6.3787) -> (-8.1464, -6.7322) centre (-8.5, -6.3787) ccw
  line L19 (6.3787, -9) -> (-6.3787, -9)
  arc A23 (-6.7322, -8.1464) -> (-6.3787, -9) centre (-6.3787, -8.5) ccw
  line L20 (-6.7322, -8.1464) -> (-0.7071, -2.1213)
  arc A24 (0.7071, -2.1213) -> (-0.7071, -2.1213) centre (0, -2.8284) ccw
  line L21 (0.7071, -2.1213) -> (6.7322, -8.1464)
  arc A25 (6.3787, -9) -> (6.7322, -8.1464) centre (6.3787, -8.5) ccw
  arc A26 (9.266, 38.142) -> (7.6383, 38.7303) centre (7.8393, 36.7404) ccw
  line L22 (9.266, 38.142) -> (19.2664, 27.9622)
  arc A27 (17.8415, 24.5606) -> (19.2664, 27.9622) centre (17.8397, 26.5606) ccw
  line L23 (17.8415, 24.5606) -> (-17.871, 24.5283)
  arc A28 (-19.3052, 27.9241) -> (-17.871, 24.5283) centre (-17.8728, 26.5283) ccw
  line L24 (-19.3052, 27.9241) -> (-9.3455, 38.1438)
  arc A29 (-7.7103, 38.7376) -> (-9.3455, 38.1438) centre (-7.9132, 36.7479) ccw
  arc A30 (-7.7103, 38.7376) -> (7.6383, 38.7303) centre (0, 114.3455) ccw
  line L25 (41.7895, -17.0192) -> (61.9965, -63.6935)
  arc A31 (55.3948, -68.0303) -> (61.9965, -63.6935) centre (58.3475, -65.3318) ccw
  line L26 (55.3948, -68.0303) -> (23.5953, -33.2362)
  arc A32 (23.7067, -29.0729) -> (23.5953, -33.2362) centre (25.8097, -31.2123) ccw
  line L27 (23.7067, -29.0729) -> (36.9334, -16.0716)
  arc A33 (41.7895, -17.0192) -> (36.9334, -16.0716) centre (39.0364, -18.2111) ccw
  line L28 (5, -97.464) -> (5, -58.6595)
  arc A34 (7, -56.6595) -> (5, -58.6595) centre (7, -58.6595) ccw
  line L29 (7, -56.6595) -> (10.473, -56.6595)
  arc A35 (14.3032, -58.4456) -> (10.473, -56.6595) centre (10.473, -61.6595) ccw
  line L30 (14.3032, -58.4456) -> (34.3305, -82.3132)
  arc A36 (35.4243, -86.3954) -> (34.3305, -82.3132) centre (30.5003, -85.5271) ccw
  line L31 (35.4243, -86.3954) -> (32.7648, -101.4781)
  arc A37 (26.9725, -105.5339) -> (32.7648, -101.4781) centre (27.8408, -100.6098) ccw
  line L32 (26.9725, -105.5339) -> (9.1318, -102.3881)
  arc A38 (5, -97.464) -> (9.1318, -102.3881) centre (10, -97.464) ccw
  arc A39 (-40.9054, 16.7074) -> (-37.3489, 15.6517) centre (-38.8619, 17.0732) ccw
  line L33 (-40.9054, 16.7074) -> (-46.7322, 29.5993)
  arc A40 (-44.339, 36.0244) -> (-46.7322, 29.5993) centre (-42.0339, 31.5075) ccw
  arc A41 (-44.339, 36.0244) -> (-34.6129, 45.4956) centre (-56.2565, 57.9923) ccw
  arc A42 (-28.1234, 47.5076) -> (-34.6129, 45.4956) centre (-30.28, 42.9921) ccw
  line L34 (-28.1234, 47.5076) -> (-14.9942, 41.2515)
  arc A43 (-14.46, 38.0146) -> (-14.9942, 41.2515) centre (-15.8549, 39.4469) ccw
  line L35 (-14.46, 38.0146) -> (-37.3489, 15.6517)
  arc A44 (-61.9967, -63.6938) -> (-55.4143, -68.0759) centre (-58.3695, -65.3802) ccw
  line L36 (-61.9967, -63.6938) -> (-41.8922, -17.2564)
  arc A45 (-36.246, -16.5772) -> (-41.8922, -17.2564) centre (-38.8636, -18.6251) ccw
  line L37 (-36.246, -16.5772) -> (-23.6374, -29.1331)
  arc A46 (-23.5625, -33.2372) -> (-23.6374, -29.1331) centre (-25.7596, -31.2246) ccw
  line L38 (-23.5625, -33.2372) -> (-55.4143, -68.0759)
  arc A47 (-46.7294, -108.889) -> (-25.7561, -114.8285) centre (-25.7561, -74.8285) ccw
  line L39 (-25.7561, -114.8285) -> (22.9214, -114.8285)
  arc A48 (22.9214, -114.8285) -> (44.7852, -108.3244) centre (22.9214, -74.8285) ccw
  arc A49 (72.6915, -102.3213) -> (44.7852, -108.3244) centre (66.5604, -141.6847) ccw
  arc A50 (72.6915, -102.3213) -> (70.4711, -73.2) centre (75, -87.5) ccw
  line L40 (70.4711, -73.2) -> (50.5773, -27.2494)
  arc A51 (51.0282, 29.3922) -> (50.5773, -27.2494) centre (114.8154, 0.5617) ccw
  line L41 (51.0282, 29.3922) -> (70.7852, 73.1043)
  arc A52 (70.7852, 73.1043) -> (60.1979, 89.9288) centre (75, 87.5) ccw
  arc A53 (35.9657, 79.8952) -> (60.1979, 89.9288) centre (-0.31, 201.7835) ccw
  line L42 (35.9657, 79.8952) -> (2.1827, 93.0889)
  arc A54 (2.1827, 93.0889) -> (-2.1423, 93.1045) centre (0, 87.5) ccw
  line L43 (-2.1423, 93.1045) -> (-36.9275, 79.8081)
  arc A55 (-60.2098, 89.9999) -> (-36.9275, 79.8081) centre (2.2046, 200.8918) ccw
  arc A56 (-60.2098, 89.9999) -> (-70.7852, 73.1043) centre (-75, 87.5) ccw
  line L44 (-70.7852, 73.1043) -> (-51.0282, 29.3922)
  arc A57 (-50.5773, -27.2494) -> (-51.0282, 29.3922) centre (-114.8154, 0.5617) ccw
  line L45 (-50.5773, -27.2494) -> (-70.4711, -73.2)
  arc A58 (-70.4711, -73.2) -> (-73.7447, -102.4474) centre (-75, -87.5) ccw
  arc A59 (-46.7294, -108.889) -> (-73.7447, -102.4474) centre (-70.0264, -146.7235) ccw
  arc A60 (-38.7303, -7.6383) -> (-38.142, -9.266) centre (-36.7404, -7.8393) ccw
  arc A61 (-38.7303, -7.6383) -> (-38.7376, 7.7103) centre (-114.3455, 0) ccw
  arc A62 (-38.1438, 9.3455) -> (-38.7376, 7.7103) centre (-36.7479, 7.9132) ccw
  line L46 (-38.1438, 9.3455) -> (-27.9241, 19.3052)
  arc A63 (-24.5283, 17.871) -> (-27.9241, 19.3052) centre (-26.5283, 17.8728) ccw
  line L47 (-24.5283, 17.871) -> (-24.5606, -17.8415)
  arc A64 (-27.9622, -19.2664) -> (-24.5607, -17.8415) centre (-26.5606, -17.8397) ccw
  line L48 (-27.9622, -19.2664) -> (-38.142, -9.266)
  arc A65 (-10.473, -56.6595) -> (-14.3032, -58.4456) centre (-10.473, -61.6595) ccw
  line L49 (-10.473, -56.6595) -> (-7, -56.6595)
  arc A66 (-5, -58.6595) -> (-7, -56.6595) centre (-7, -58.6595) ccw
  line L50 (-5, -58.6595) -> (-5, -97.464)
  arc A67 (-9.1318, -102.3881) -> (-5, -97.464) centre (-10, -97.464) ccw
  line L51 (-9.1318, -102.3881) -> (-26.9725, -105.5339)
  arc A68 (-32.7648, -101.4781) -> (-26.9725, -105.5339) centre (-27.8408, -100.6098) ccw
  line L52 (-32.7648, -101.4781) -> (-35.4243, -86.3954)
  arc A69 (-34.3305, -82.3132) -> (-35.4243, -86.3954) centre (-30.5003, -85.5271) ccw
  line L53 (-34.3305, -82.3132) -> (-14.3032, -58.4456)
  arc A70 (37.4337, 15.5639) -> (40.6601, 16.1647) centre (38.8376, 16.9884) ccw
  line L54 (37.4337, 15.5639) -> (14.6425, 38.0264)
  arc A71 (15.1963, 41.2612) -> (14.6425, 38.0264) centre (16.0464, 39.4508) ccw
  line L55 (15.1963, 41.2612) -> (28.3187, 47.4234)
  arc A72 (34.7856, 45.3775) -> (28.3187, 47.4234) centre (30.444, 42.8975) ccw
  arc A73 (34.7856, 45.3775) -> (44.4886, 35.8486) centre (56.4937, 57.7776) ccw
  arc A74 (46.6438, 29.4035) -> (44.4886, 35.8486) centre (42.0875, 31.4628) ccw
  line L56 (46.6438, 29.4035) -> (40.6601, 16.1647)
  line L57 (-6.3787, 9) -> (6.3787, 9)
  arc A75 (6.7322, 8.1464) -> (6.3787, 9) centre (6.3787, 8.5) ccw
  line L58 (6.7322, 8.1464) -> (0.7071, 2.1213)
  arc A76 (-0.7071, 2.1213) -> (0.7071, 2.1213) centre (0, 2.8284) ccw
  line L59 (-0.7071, 2.1213) -> (-6.7322, 8.1464)
  arc A77 (-6.3787, 9) -> (-6.7322, 8.1464) centre (-6.3787, 8.5) ccw
  circle A78 centre (-40.65, 60) radius 2.15
  line L60 (47.15, 42.4858) -> (47.15, 67.561)
  arc A79 (49.4611, 71.7764) -> (47.15, 67.561) centre (52.15, 67.561) ccw
  line L61 (49.4611, 71.7764) -> (57.5607, 76.943)
  arc A80 (64.8173, 70.6939) -> (57.5607, 76.943) centre (60.2496, 72.7276) ccw
  line L62 (64.8173, 70.6939) -> (51.1653, 40.0309)
  arc A81 (49.5538, 39.7214) -> (51.1653, 40.0309) centre (50.2517, 40.4376) ccw
  line L63 (49.5538, 39.7214) -> (47.4521, 41.7697)
  arc A82 (47.15, 42.4858) -> (47.4521, 41.7697) centre (48.15, 42.4858) ccw
  circle A83 centre (40.65, 60) radius 2.15
  circle A84 centre (-40.65, 50) radius 2.15
  arc A85 (-57.5607, 76.943) -> (-64.8173, 70.6939) centre (-60.2496, 72.7276) ccw
  line L64 (-57.5607, 76.943) -> (-49.4611, 71.7764)
  arc A86 (-47.15, 67.561) -> (-49.4611, 71.7764) centre (-52.15, 67.561) ccw
  line L65 (-47.15, 67.561) -> (-47.15, 42.4858)
  arc A87 (-47.4521, 41.7697) -> (-47.15, 42.4858) centre (-48.15, 42.4858) ccw
  line L66 (-47.4521, 41.7697) -> (-49.5538, 39.7214)
  arc A88 (-51.1653, 40.0309) -> (-49.5538, 39.7214) centre (-50.2517, 40.4376) ccw
  line L67 (-51.1653, 40.0309) -> (-64.8173, 70.6939)
  circle A89 centre (40.65, 50) radius 2.15
  circle A90 centre (10, -10) radius 1.5
  circle A91 centre (-10, -10) radius 1.5
  circle A92 centre (10, 10) radius 1.5
  circle A93 centre (-10, 10) radius 1.5
  dimension "d174" = 3
  dimension "d177" = -20
  dimension "d178" = 20
  measures "d174" diameter of A90
hole "Furo1" at (-10, 10, 2) at (10, 10, 2) at (10, -10, 2) at (-10, -10, 2) direction (0, 0, -1) diameter 3.3 end through all countersink diameter 6 countersink angle 57